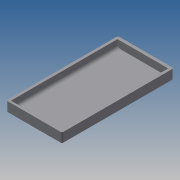
# Autodesk Inventor part: Case
Saved by Autodesk Inventor 2014 (Build 180170000, 170)
## iProperties
Created: 2014-04-28
Part Number: Case
Material: Generic
Document SubType Name: Modeling
Designer: 1770749
Density: 1 g/cm^3
Appearance: Default
Author: 1770749
Autodesk Inventor part; units mm, degrees
ref_plane "YZ Plane" through (0, 0, 0) normal (1, 0, 0) x (0, 1, 0)
ref_plane "XZ Plane" through (0, 0, 0) normal (0, 1, 0) x (-1, 0, 0)
ref_plane "XY Plane" through (0, 0, 0) normal (0, 0, 1) x (1, 0, 0)
sketch "Sketch1" plane through (0, 0, 0) normal (0, 0, 1) x (1, 0, 0)
  line L0 (0, 0) -> (59.18, 0)
  line L1 (59.18, 0) -> (59.18, 124.44)
  line L2 (59.18, 124.44) -> (0, 124.44)
  line L3 (0, 124.44) -> (0, 0)
  dimension "d2" = 124.44
  dimension "d3" = 59.18
  constraints: 8 end point, 2 parallel, 1 horizontal, 1 perpendicular
  measures "d2" distance of L0.end L1.end
  measures "d3" distance of L1.end L2.end
sketch "Sketch2" plane through (0, 0, 0) normal (0, 0, 1) x (1, 0, 0)
  line L0 (-3, -2.5179) -> (62.18, -2.5179)
  line L1 (62.18, -2.5179) -> (62.18, 127.9221)
  line L2 (62.18, 127.9221) -> (-3, 127.9221)
  line L3 (-3, 127.9221) -> (-3, -2.5179)
  point P0 (0, 0)
  dimension "d4" = 65.18
  dimension "d5" = 130.44
  constraints: 8 end point, 2 parallel, 1 horizontal, 1 perpendicular
  measures "d4" distance of L2.end L1.end
  measures "d5" distance of L0.end L1.end
extrude "Extrusion1" add sketch "Sketch2" against normal blind 11.5
extrude "Extrusion2" cut sketch "Sketch1" against normal blind 8.5
fillet "Fillet1" radius 2 1 edges at (62.18, 127.9221, -5.75)
fillet "Fillet2" radius 2 1 edges at (-3, 127.9221, -5.75)
fillet "Fillet3" radius 2 1 edges at (62.18, -2.5179, -5.75)
fillet "Fillet4" radius 2 1 edges at (-3, -2.5179, -5.75)
fillet "Fillet5" radius 1 8 edges at (61.5942, -1.9321, -11.5) (29.59, -2.5179, -11.5) (-2.4142, -1.9321, -11.5) (-3, 62.7021, -11.5) (-2.4142, 127.3363, -11.5) (29.59, 127.9221, -11.5) (61.5942, 127.3363, -11.5) (62.18, 62.7021, -11.5)
fillet "Fillet6" radius 3.74 1 edges at (0, 62.22, -8.5)
fillet "Fillet7" radius 3.74 1 edges at (59.18, 62.22, -8.5)
body "Solid1"
